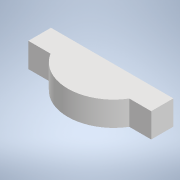
# Autodesk Inventor part: 14_base_avanti
Saved by Autodesk Inventor 2020 (Build 240168000, 168)
## iProperties
Created: 2019-10-17
Part Number: 14_base_avanti
Material: Generico
Document SubType Name: Modeling
Designer: socci
Density: 1 g/cm^3
Appearance: Default
Author: socci
Autodesk Inventor part; units mm, degrees
ref_plane "YZ Plane" through (0, 0, 0) normal (1, 0, 0) x (0, 1, 0)
ref_plane "XZ Plane" through (0, 0, 0) normal (0, 1, 0) x (-1, 0, 0)
ref_plane "XY Plane" through (0, 0, 0) normal (0, 0, 1) x (1, 0, 0)
sketch "Schizzo1" plane through (0, 0, 0) normal (0, 1, 0) x (-1, 0, 0)
  line L0 (40, -14.5) -> (-40, -14.5)
  line L1 (-40, -14.5) -> (-40, 14.5)
  line L2 (-40, 14.5) -> (40, 14.5)
  line L3 (40, 14.5) -> (40, -14.5)
  line L4 (40, -14.5) -> (-40, 14.5) construction
  line L5 (-40, -14.5) -> (40, 14.5) construction
  point P0 (0, 0)
  point P1 (0, 0)
  point P2 (0, 0)
  dimension "d0" = 29
  dimension "d15" = 80
  constraints: 12 end point, 3 midpoint, 2 parallel, 1 coincident, 1 horizontal, 1 perpendicular
  measures "d0" distance of L0.end L1.end
  measures "d15" distance of L1.end L2.end
extrude "Estrusione1" add sketch "Schizzo1" along normal blind 16
sketch "Schizzo2" plane through (0, 0, 0) normal (0, -1, 0) x (1, 0, 0)
  line L0 (40, -14.5) -> (-40, -14.5) projected
  line L1 (0, -14.5) -> (0, -15.5)
  line L2 (0, -14.5) -> (1, -14.5) construction
  circle A0 centre (0, -15.5) radius 9.5
  point P0 (0, 0)
  dimension "d9" = 1
  dimension "d10" = 90
  dimension "d11" = 19
  constraints: 4 end point, 1 centre point, 1 coincident, 1 horizontal, 1 midpoint, 1 perpendicular, 1 vertical
  measures "d9" distance of L1.start L1.end
  measures "d10" angle of L1 L2
  measures "d11" diameter of A0
extrude "Estrusione2" cut sketch "Schizzo2" against normal blind 4
sketch "Schizzo3" plane through (0, 4, 0) normal (0, -1, 0) x (1, 0, 0)
  line L0 (9.4472, -14.5) -> (-9.4472, -14.5) projected
  line L1 (0, -14.5) -> (0, -15.5)
  line L2 (0, -14.5) -> (1, -14.5) construction
  circle A0 centre (0, -15.5) radius 6
  point P0 (0, 0)
  point P1 (9.5, -24.5)
  point P2 (-9.5, -24.5)
  point P3 (-9.4472, -14.5)
  dimension "d12" = 1
  dimension "d13" = 90
  dimension "d14" = 12
  constraints: 4 end point, 1 centre point, 1 coincident, 1 horizontal, 1 perpendicular, 1 vertical, 2 other
  measures "d12" distance of L1.start L1.end
  measures "d13" angle of L1 L2
  measures "d14" diameter of A0
extrude "Estrusione3" cut sketch "Schizzo3" against normal blind 10
sketch "Schizzo5" plane through (0, 16, 0) normal (0, 1, 0) x (1, 0, 0)
  line L0 (40, 14.5) -> (-40, 14.5) projected
  line L1 (0, 14.5) -> (0, 15.5)
  line L2 (0, 14.5) -> (1, 14.5) construction
  circle A0 centre (0, 15.5) radius 30
  line L3 (40, -14.5) -> (40, 14.5) projected
  line L4 (-40, -14.5) -> (40, -14.5) projected
  line L5 (0, -14.5) -> (40, -14.5)
  line L6 (40, -14.5) -> (40, 14.5) projected
  line L7 (40, 0) -> (25.6856, 0)
  line L8 (0, -14.5) -> (-40, -14.5)
  line L9 (-40, -14.5) -> (-40, -0.3172)
  line L10 (-40, 14.5) -> (-40, -14.5) projected
  line L11 (-40, -14.5) -> (-40, -0.3172)
  line L12 (-25.4915, -0.3172) -> (-40, -0.3172)
  point P0 (0, 0)
  dimension "d16" = 1
  dimension "d17" = 90
  constraints: 16 end point, 3 collinear, 3 midpoint, 3 point on circle, 2 horizontal, 2 perpendicular, 1 centre point, 1 coincident, 1 vertical
  measures "d16" distance of L1.start L1.end
  measures "d17" angle of L2 L1
extrude "Estrusione4" cut sketch "Schizzo5" against normal blind 30 contours L3 L4 A0 L7 | L4 L9 L12 A0
